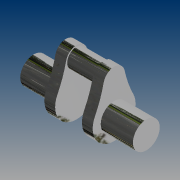
# Autodesk Inventor part: crankshaft
Saved by Autodesk Inventor 2015 (Build 190159000, 159)
## iProperties
Created: 2021-03-23
Part Number: crankshaft
Material: Silicon Nitride
Document SubType Name: Modeling
Designer: Diptanshu Das
Density: 3.18 g/cm^3
Appearance: Chrome - Polished Black
Author: Diptanshu Das
Autodesk Inventor part; units mm, degrees
ref_plane "YZ Plane" through (0, 0, 0) normal (1, 0, 0) x (0, 1, 0)
ref_plane "XZ Plane" through (0, 0, 0) normal (0, 1, 0) x (-1, 0, 0)
sketch "Sketch4" plane through (0, 0, 0) normal (1, 0, 0) x (0, 1, 0)
  arc A0 (-35.8323, 17.7778) -> (35.8323, 17.7778) centre (0, 0) ccw
  arc A1 (19.5449, 64.2424) -> (-19.5449, 64.2424) centre (0, 60) ccw
  arc A2 (-35.8323, 17.7778) -> (-19.5449, 64.2424) centre (-214.9935, 106.6667) ccw
  arc A3 (19.5449, 64.2424) -> (35.8323, 17.7778) centre (214.9935, 106.6667) ccw
  dimension "d13" = 80
  dimension "d14" = 40
  dimension "d15" = 60
  dimension "d16" = 200
  dimension "d17" = 200
  constraints: 8 point on circle, 4 centre point, 4 tangent, 1 coincident, 1 vertical alignment
  measures "d13" diameter of A0
  measures "d14" diameter of A1
  measures "d15" distance of A0.centre A1.centre
  measures "d16" radius of A2
  measures "d17" radius of A3
extrude "Extrusion4" add sketch "Sketch4" along normal blind 20
sketch "Sketch5" plane through (20, 0, 0) normal (1, 0, 0) x (0, 0, -1)
  arc A0 (-17.7778, -35.8323) -> (-17.7778, 35.8323) centre (0, 0) ccw projected
  circle A1 centre (0, 0) radius 25
  dimension "d20" = 50
  constraints: 1 centre point, 1 coincident
  measures "d20" diameter of A1
extrude "Extrusion5" add sketch "Sketch5" along normal blind 60
sketch "Sketch6" plane through (0, 0, 0) normal (-1, 0, 0) x (0, 0, 1)
  arc A0 (64.2424, -19.5449) -> (64.2424, 19.5449) centre (60, 0) ccw projected
  circle A1 centre (60, 0) radius 17.5
  dimension "d23" = 35
  constraints: 1 centre point, 1 coincident
  measures "d23" diameter of A1
extrude "Extrusion6" add sketch "Sketch6" along normal blind 50
ref_plane "Work Plane2" through (-25, 0, 60) normal (-1, 0, 0) x (0, 0, 1)
mirror "Mirror3" about plane through (-25, 0, 60) normal (-1, 0, 0) of "Extrusion4"
mirror "Mirror4" about plane through (-25, 0, 60) normal (-1, 0, 0) of "Extrusion5"
body "Solid2"
